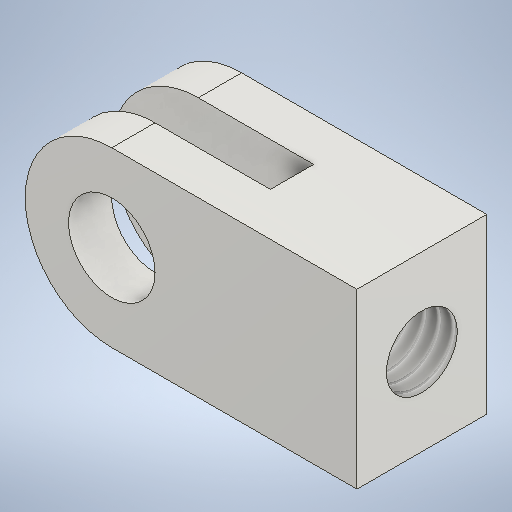
# Autodesk Inventor part: 30 - Eccentric Rod 2
Saved by Autodesk Inventor 2025.2 (Build 292293000, 293)
## iProperties
Created: 2025-07-30
Part Number: 30 - Eccentric Rod 2
Material: Steel AISI 1020 107 HR
Document SubType Name: Modeling
Designer: bless
Density: 7.87 g/cm^3
Appearance: Steel
Author: bless
Autodesk Inventor part; units mm, degrees
ref_plane "YZ Plane" through (0, 0, 0) normal (1, 0, 0) x (0, 1, 0)
ref_plane "XZ Plane" through (0, 0, 0) normal (0, 1, 0) x (-1, 0, 0)
ref_plane "XY Plane" through (0, 0, 0) normal (0, 0, 1) x (1, 0, 0)
sketch "Sketch1" plane through (0, 0, 0) normal (0, 0, 1) x (1, 0, 0)
  line L0 (0, 0) -> (8.5, 0)
  line L1 (8.5, 0) -> (8.5, 6)
  line L2 (8.5, 6) -> (0, 6)
  line L3 (0, 6) -> (0, 0) construction
  circle A0 centre (0, 3) radius 3
  circle A1 centre (0, 3) radius 1.5
  dimension "d0" = 8.5
  dimension "d1" = 6
  dimension "d2" = 3
  constraints: 8 end point, 2 parallel, 1 centre point, 1 coincident, 1 horizontal, 1 midpoint, 1 perpendicular, 3 other
  measures "d0" distance of L2.end L1.end
  measures "d1" distance of L1.end L0.end
  measures "d2" diameter of A1
extrude "Extrusion1" add sketch "Sketch1" against normal blind 4.5
sketch "Sketch2" plane through (0, 6, 0) normal (0, 1, 0) x (1, 0, 0)
  line L0 (8.5, 0) -> (8.5, 4.5) projected
  line L1 (0, 0) -> (0, 0) projected
  line L2 (0, 0) -> (0, 4.5) projected
  line L3 (0, 4.5) -> (0, 4.5) projected
  line L4 (0, 0) -> (0, 4.5) projected
  line L5 (-3, 0) -> (-3, 4.5) projected
  line L6 (-3, 0) -> (0, 0) projected
  line L7 (0, 4.5) -> (-3, 4.5) projected
  line L8 (-3, 1.5) -> (4, 1.5)
  line L9 (4, 1.5) -> (4, 3)
  line L10 (4, 3) -> (-3, 3)
  line L11 (-3, 3) -> (-3, 1.5)
  point P0 (4, 2.25)
  point P1 (8.5, 2.25)
  dimension "d7" = 1.5
  dimension "d8" = 7
  constraints: 8 end point, 2 midpoint, 2 parallel, 1 horizontal, 1 horizontal alignment, 1 perpendicular, 1 point on line
  measures "d7" distance of L8.end L9.end
  measures "d8" distance between parallel lines of L5 L9
extrude "Extrusion2" cut sketch "Sketch2" against normal through all contours L8 L5 L10 L2 | L2 L10 L9 L8
sketch "Sketch3" plane through (8.5, 0, 0) normal (1, 0, 0) x (0, 0, -1)
  line L0 (4.5, 6) -> (4.5, 0) projected
  line L1 (0, 6) -> (4.5, 6) projected
  point P0 (2.25, 3)
  dimension "d11" = 3
  dimension "d12" = 2.25
  measures "d11" distance from line of point (2.25, 3) L1
  measures "d12" distance from line of point (2.25, 3) L0
hole "Hole1" at (8.5, 3, -2.25) direction (-1, 0, 0) diameter 2.459 depth 5.5 tip angle 118 thread size "M3x0.5" class "6H" standard "ANSI Metric M Profile"
body "Solid1"
